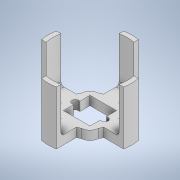
# Autodesk Inventor part: mirror_mount_empty
Saved by Autodesk Inventor 2020 (Build 240168000, 168)
## iProperties
Created: 2024-03-15
Part Number: mirror_mount_empty
Material: Типовые
Document SubType Name: Modeling
Designer: 4s
Density: 1 g/cm^3
Appearance: По умолчанию
Author: 4s
Autodesk Inventor part; units mm, degrees
ref_plane "YZ Plane" through (0, 0, 0) normal (1, 0, 0) x (0, 1, 0)
ref_plane "XZ Plane" through (0, 0, 0) normal (0, 1, 0) x (-1, 0, 0)
ref_plane "XY Plane" through (0, 0, 0) normal (0, 0, 1) x (1, 0, 0)
sketch "Эскиз1" plane through (0, 0, 0) normal (0, 1, 0) x (-1, 0, 0)
  line L0 (8.9, -8.9) -> (-8.9, -8.9)
  line L1 (-8.9, -8.9) -> (-8.9, -2.1)
  line L2 (-8.9, 8.9) -> (8.9, 8.9)
  line L3 (8.9, 8.9) -> (8.9, 2.1)
  line L4 (0, 0) -> (0, -10.3494) construction
  line L5 (0, 0) -> (-17.6402, 0) construction
  circle A0 centre (10, 0) radius 0.9 construction
  circle A1 centre (-10, 0) radius 0.9 construction
  arc A2 (10, -2.1) -> (10, 2.1) centre (10, 0) ccw
  line L6 (10, -2.1) -> (8.9, -2.1)
  line L7 (10, 2.1) -> (8.9, 2.1)
  line L8 (8.9, -2.1) -> (8.9, -8.9)
  line L9 (8.9, 2.1) -> (8.9, -2.1) construction
  circle A3 centre (-10, 0) radius 0.9 construction
  arc A4 (-10, 2.1) -> (-10, -2.1) centre (-10, 0) ccw
  line L10 (-10, -2.1) -> (-8.9, -2.1)
  line L11 (-10, 2.1) -> (-8.9, 2.1)
  line L12 (-8.9, -2.1) -> (-8.9, 2.1) construction
  line L13 (-8.9, 2.1) -> (-8.9, 8.9)
  circle A5 centre (0, 0) radius 15
  arc A6 (-24.4949, -5) -> (-24.4949, 5) centre (0, 0) ccw construction
  line L14 (-14.1421, -5) -> (-27.55, -5)
  line L15 (-27.55, 5) -> (-14.1421, 5)
  arc A7 (-27.55, -5) -> (-27.55, 5) centre (0, 0) ccw construction
  arc A8 (-24.4949, 5) -> (-24.4949, -5) centre (0, 0) ccw
  arc A9 (-27.55, 5) -> (-27.55, -5) centre (0, 0) ccw
  line L16 (14.1421, -5) -> (27.55, -5)
  line L17 (27.55, 5) -> (14.1421, 5)
  arc A10 (24.4949, -5) -> (24.4949, 5) centre (0, 0) ccw
  arc A11 (27.55, -5) -> (27.55, 5) centre (0, 0) ccw
  line L18 (0, 0) -> (-17.6777, -17.6777) construction
  line L19 (0, 0) -> (25, 0) construction
  line L20 (-5, -14.1421) -> (-5, -27.55)
  line L21 (5, -27.55) -> (5, -14.1421)
  arc A12 (-5, -24.4949) -> (5, -24.4949) centre (0, 0) ccw
  arc A13 (-5, -27.55) -> (5, -27.55) centre (0, 0) ccw
  arc A14 (5, 24.4949) -> (-5, 24.4949) centre (0, 0) ccw
  line L22 (-5, 14.1421) -> (-5, 27.55)
  arc A15 (5, 27.55) -> (-5, 27.55) centre (0, 0) ccw
  line L23 (5, 27.55) -> (5, 14.1421)
  arc A16 (-13.0635, -7.3719) -> (-7.3719, -13.0635) centre (-7.0711, -7.0711) ccw
  arc A17 (7.3719, -13.0635) -> (13.0635, -7.3719) centre (7.0711, -7.0711) ccw
  arc A18 (-7.3719, 13.0635) -> (-13.0635, 7.3719) centre (-7.0711, 7.0711) ccw
  arc A19 (13.0635, 7.3719) -> (7.3719, 13.0635) centre (7.0711, 7.0711) ccw
  point P0 (17.6402, 0)
  point P1 (0, -17.6402)
  point P2 (0, 17.6402)
  point P3 (0, 25)
  point P4 (-13.0635, 7.3719)
  point P5 (-7.3719, 13.0635)
  point P6 (13.0635, -7.3719)
  point P7 (7.3719, -13.0635)
  point P8 (7.3719, 13.0635)
  point P9 (13.0635, 7.3719)
  dimension "d0" = 17.8
  dimension "d1" = 17.8
  dimension "d2" = 1.8
  dimension "d3" = 20
  dimension "d4" = 4.2
  dimension "d5" = 30
  dimension "d15" = 50
  dimension "d17" = 10
  dimension "d18" = 3
  dimension "d19" = 135
  dimension "d22" = 12
  dimension "d23" = 10
  constraints: 48 end point, 40 symmetric about line, 36 point on circle, 20 centre point, 12 parallel, 10 point on line, 8 coincident, 4 horizontal, 3 perpendicular, 1 equal length, 1 tangent, 1 vertical, 15 other
  measures "d0" distance between parallel lines of L1 L3
  measures "d1" distance between parallel lines of L2 L0
  measures "d2" diameter of A0
  measures "d3" distance of A1.centre A0.centre
  measures "d4" diameter of A2
  measures "d5" diameter of A5
  measures "d15" diameter of A6
  measures "d17" distance between parallel lines of L15 L14
  measures "d18" radial gap between concentric circles of A6 A7
  measures "d19" angle of L18 L19
  measures "d22" diameter of A16
  measures "d23" distance of A16.centre L4.start
extrude "Выдавливание1" add sketch "Эскиз1" along normal blind 6 contours A5 | A5 L17 A10 L16 | A5 A19 | A17 A5 | A5 L22 A14 L23 | L21 A12 L20 A5 | A5 A18 | A16 A5 | A5 L14 A8 L15
sketch "Эскиз2" plane through (0, 0, 0) normal (0, 1, 0) x (-1, 0, 0)
  arc A0 (-13.0635, 7.3719) -> (-14.1421, 5) centre (0, 0) ccw construction
  line L0 (8.9, -2.1) -> (8.9, -8.9) construction
  line L1 (8.9, -8.9) -> (-8.9, -8.9) construction
  line L2 (-8.9, -8.9) -> (-8.9, -2.1) construction
  line L3 (-8.9, -2.1) -> (-10, -2.1) construction
  arc A1 (-10, 2.1) -> (-10, -2.1) centre (-10, 0) ccw construction
  line L4 (-10, 2.1) -> (-8.9, 2.1) construction
  line L5 (-8.9, 2.1) -> (-8.9, 8.9) construction
  line L6 (-8.9, 8.9) -> (8.9, 8.9) construction
  line L7 (8.9, 8.9) -> (8.9, 2.1) construction
  line L8 (8.9, 2.1) -> (10, 2.1) construction
  arc A2 (10, -2.1) -> (10, 2.1) centre (10, 0) ccw construction
  line L9 (10, -2.1) -> (8.9, -2.1) construction
  circle A3 centre (14.713, -5.4) radius 1.4
  line L10 (0, 0) -> (0, -15) construction
  circle A4 centre (-14.713, -5.4) radius 1.4
  arc A5 (12.5706, -3.3) -> (16.8554, -3.3) centre (14.713, -5.4) ccw
  arc A6 (-16.8554, -3.3) -> (-12.5706, -3.3) centre (-14.713, -5.4) ccw
  line L11 (14.713, -5.4) -> (14.713, -3.3) construction
  line L12 (16.8554, -3.3) -> (12.5706, -3.3)
  line L13 (-16.8554, -3.3) -> (-12.5706, -3.3)
  arc A7 (-5, 14.1421) -> (-7.3719, 13.0635) centre (0, 0) ccw projected
  line L14 (-5, -14.1421) -> (-5, -24.4949) projected
  arc A8 (-5, -24.4949) -> (5, -24.4949) centre (0, 0) ccw projected
  line L15 (5, -24.4949) -> (5, -14.1421) projected
  line L16 (14.1421, -5) -> (24.4949, -5) projected
  arc A9 (24.4949, -5) -> (24.4949, 5) centre (0, 0) ccw projected
  line L17 (24.4949, 5) -> (14.1421, 5) projected
  arc A10 (7.3719, 13.0635) -> (5, 14.1421) centre (0, 0) ccw projected
  line L18 (5, 14.1421) -> (5, 24.4949) projected
  arc A11 (5, 24.4949) -> (-5, 24.4949) centre (0, 0) ccw projected
  line L19 (-5, 24.4949) -> (-5, 14.1421) projected
  arc A12 (14.1421, 5) -> (13.0635, 7.3719) centre (0, 0) ccw projected
  line L20 (-14.1421, 5) -> (-24.4949, 5) projected
  arc A13 (-24.4949, 5) -> (-24.4949, -5) centre (0, 0) ccw projected
  line L21 (-24.4949, -5) -> (-14.1421, -5) projected
  arc A14 (-14.1421, -5) -> (-13.0635, -7.3719) centre (0, 0) ccw projected
  arc A15 (-13.0635, -7.3719) -> (-7.3719, -13.0635) centre (-7.0711, -7.0711) ccw projected
  arc A16 (-7.3719, -13.0635) -> (-5, -14.1421) centre (0, 0) ccw projected
  arc A17 (5, -14.1421) -> (7.3719, -13.0635) centre (0, 0) ccw projected
  arc A18 (7.3719, -13.0635) -> (13.0635, -7.3719) centre (7.0711, -7.0711) ccw projected
  arc A19 (13.0635, -7.3719) -> (14.1421, -5) centre (0, 0) ccw projected
  arc A20 (13.0635, 7.3719) -> (7.3719, 13.0635) centre (7.0711, 7.0711) ccw projected
  arc A21 (-7.3719, 13.0635) -> (-13.0635, 7.3719) centre (-7.0711, 7.0711) ccw projected
  dimension "d8" = 2.8
  dimension "d9" = 3.3
  dimension "d10" = 29.426
  dimension "d11" = 6
  dimension "d14" = 2.1
  constraints: 8 end point, 5 point on circle, 4 centre point, 4 symmetric about line, 2 vertical, 1 coincident, 1 horizontal, 1 midpoint, 2 other
  measures "d8" diameter of A3
  measures "d9" distance from line of L9 A3.centre
  measures "d10" distance of A4.centre A3.centre
  measures "d11" diameter of A5
  measures "d14" distance of L11.start L11.end
extrude "Выдавливание2" [suppressed]
extrude "Выдавливание3" add sketch "Эскиз1" along normal blind 36 contours L17 A11 L16 A10 | A14 L22 A15 L23 | L21 A13 L20 A12 | A8 L14 A9 L15
fillet "Сопряжение1" radius 2 4 edges at (0, 6, -25) (25, 6, 0) (-25, 6, 0) (0, 6, 25)
